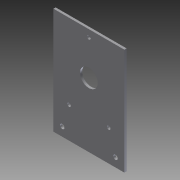
# Autodesk Inventor part: window motor plate
Saved by Autodesk Inventor 2011 SP1 (Build 150282100, 282)
## iProperties
Created: 2012-01-19
Part Number: window motor plate
Document SubType Name: Modeling
Designer: Christopher
Density: 1 g/cm^3
Author: Christopher
Autodesk Inventor part; units mm, degrees
ref_plane "YZ Plane" through (0, 0, 0) normal (1, 0, 0) x (0, 1, 0)
ref_plane "XZ Plane" through (0, 0, 0) normal (0, 1, 0) x (-1, 0, 0)
ref_plane "XY Plane" through (0, 0, 0) normal (0, 0, 1) x (1, 0, 0)
sketch "Sketch1" plane through (0, 0, 0) normal (0, 0, 1) x (1, 0, 0)
  line L0 (0, 0) -> (101.6, 0)
  line L1 (101.6, 0) -> (101.6, 152.4)
  line L2 (101.6, 152.4) -> (0, 152.4)
  line L3 (0, 152.4) -> (0, 0)
  point P0 (22.4155, 44.45)
  point P1 (79.1845, 44.45)
  point P2 (50.8, 141.9352)
  point P3 (50.8, 93.6625)
  point P4 (12.7, 12.7)
  point P5 (88.9, 12.7)
  dimension "d0" = 152.4
  dimension "d1" = 101.6
  dimension "d2" = 44.45
  dimension "d3" = 49.2125
  dimension "d4" = 97.4852
  dimension "d5" = 56.769
  dimension "d6" = 28.3845
  dimension "d7" = 12.7
  dimension "d8" = 12.7
  dimension "d9" = 12.7
  dimension "d10" = 50.8
  constraints: 8 end point, 2 horizontal alignment, 2 parallel, 1 horizontal, 1 perpendicular, 1 vertical alignment
  measures "d0" distance of L2.end L0.start
  measures "d1" distance of L0.start L0.end
  measures "d2" distance from line of L0 point (22.416, 44.45)
  measures "d3" vertical distance of point (50.8, 93.663) point (22.416, 44.45)
  measures "d4" vertical distance of point (50.8, 141.935) point (22.416, 44.45)
  measures "d5" distance of point (22.416, 44.45) point (79.184, 44.45)
  measures "d6" horizontal distance of point (50.8, 93.663) point (79.184, 44.45)
  measures "d7" distance from line of L0 point (12.7, 12.7)
  measures "d8" distance from line of L3 point (12.7, 12.7)
  measures "d9" distance from line of L1 point (88.9, 12.7)
  measures "d10" distance from line of L3 point (50.8, 93.663)
extrude "Extrusion1" add sketch "Sketch1" against normal blind 3.175
hole "Hole1" at (22.4155, 44.45, 0) at (79.1845, 44.45, 0) at (50.8, 141.9352, 0) direction (0, 0, -1) diameter 5.0038 depth 25.4 tip angle 118
hole "Hole2" at (12.7, 12.7, 0) at (88.9, 12.7, 0) direction (0, 0, -1) diameter 6.35 depth 25.4 tip angle 118
hole "Hole3" at (50.8, 93.6625, 0) direction (0, 0, -1) diameter 25.4 depth 25.4 tip angle 118
body "Solid1"
